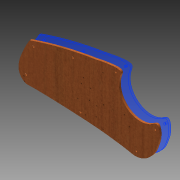
# Autodesk Inventor part: mountingBase02
Saved by Autodesk Inventor 2013 (Build 170138000, 138)
## iProperties
Created: 2014-04-26
Part Number: mountingBase02
Material: Wood (Cherry)
Document SubType Name: Modeling
Designer: Nano
Density: 0.5 g/cm^3
Mass: 26.2829 g
Surface Area: 352.098 cm^2
Volume: 52.5659 cm^3
Author: Nano
Autodesk Inventor part; units mm, degrees
ref_plane "YZ Plane" through (0, 0, 0) normal (1, 0, 0) x (0, 1, 0)
ref_plane "XZ Plane" through (0, 0, 0) normal (0, 1, 0) x (-1, 0, 0)
ref_plane "XY Plane" through (0, 0, 0) normal (0, 0, 1) x (1, 0, 0)
sketch "Sketch1" plane through (0, 0, 0) normal (0, 0, 1) x (1, 0, 0)
  circle A0 centre (22.4774, 26.9707) radius 1.5875
  circle A1 centre (125.529, -53.0458) radius 1.5875
  circle A2 centre (-41.4513, 10.4793) radius 1.5875
  circle A3 centre (-53.6193, -34.8433) radius 1.5875
  circle A4 centre (92.0523, 41.3343) radius 1.5875
  circle A5 centre (156.384, -7.2553) radius 1.5875
  circle A6 centre (34.8781, -43.685) radius 1.5875
  spline S0 degree 4 poles (-47.5552, 16.3255) (-56.6287, 2.113) (-58.2297, -5.7038) (-64.6, -14.5986) (-66.079, -30.6977) (-65.3382, -34.7532) (-63.7847, -39.1481) (-60.7246, -43.61) (-57.2762, -46.3652) (-54.2619, -47.5537) (-52.1718, -47.8438) knots 0 0 0 0 0 0.364781 0.475074 0.575005 0.66288 0.74023 0.816344 1 1 1 1 1
  spline S1 degree 2 poles (58.7626, 42.8458) (4.2199, 34.129) (-47.5552, 16.3255) knots 0 0 0 1 1 1
  spline S2 degree 4 poles (99.6942, 39.5117) (100.5315, 41.9337) (102.2753, 45.9487) (95.6149, 49.3825) (84.6696, 47.2004) (75.6939, 46.6412) (58.7626, 42.8458) knots 0 0 0 0 0 0.302315 0.43713 1 1 1 1 1
  arc A7 (99.6942, 39.5117) -> (153.3806, -0.867) centre (132.2899, 26.9707) ccw
  spline S3 degree 4 poles (-52.1718, -47.8438) (-36.534, -47.2807) (-10.4713, -48.0839) (24.7021, -49.5616) (67.2238, -52.2682) (90.8101, -55.4619) (116.0619, -59.11) (123.6331, -61.9612) (134.6517, -59.1206) (140.3653, -56.3824) (147.0584, -51.569) (152.6757, -44.8659) (156.5758, -39.5192) (161.1474, -26.3914) (163.713, -18.7298) (163.826, -8.1408) (162.8833, -4.127) (161.13, 0.717) (158.3924, 2.1696) (155.7666, 0.7307) (153.3806, -0.867) knots 0 0 0 0 0 0.199945 0.282515 0.361523 0.429862 0.488285 0.536529 0.578018 0.619243 0.659616 0.703917 0.750178 0.797252 0.841669 0.879197 0.910001 0.934907 1 1 1 1 1
  point P0 (-58.1503, -3.4556)
  point P1 (-61.848, -12.1317)
  point P2 (-64.9126, -22.073)
  point P3 (-65.6993, -31.3231)
  point P4 (-64.9927, -35.4369)
  point P5 (-63.5229, -39.1631)
  point P6 (-61.3341, -42.4183)
  point P7 (-58.5466, -45.0642)
  point P8 (-55.3853, -46.9262)
  point P9 (4.7943, 31.828)
  point P10 (100.8596, 43.7793)
  point P11 (100.1635, 46.1522)
  point P12 (97.4552, 47.5466)
  point P13 (92.3442, 47.958)
  point P14 (84.3045, 47.329)
  point P15 (-26.9279, -47.7688)
  point P16 (3.833, -48.7885)
  point P17 (37.204, -50.4527)
  point P18 (68.9137, -52.842)
  point P19 (96.8664, -56.38)
  point P20 (117.598, -59.9719)
  point P21 (125.9833, -60.7612)
  point P22 (134.5494, -58.8078)
  point P23 (140.484, -56.0059)
  point P24 (146.5961, -51.4174)
  point P25 (152.0146, -45.51)
  point P26 (156.0745, -39.2339)
  point P27 (160.8814, -27.0309)
  point P28 (163.3993, -16.4807)
  point P29 (163.3985, -7.1763)
  point P30 (162.4894, -3.2093)
  point P31 (161.1531, -0.4019)
  point P32 (159.4932, 1.023)
  point P33 (157.3679, 1.1626)
  constraints: 8 centre point, 2 point on circle, 42 other
extrude "Extrusion1" add sketch "Sketch1" against normal blind 3.175
body "Solid1"
